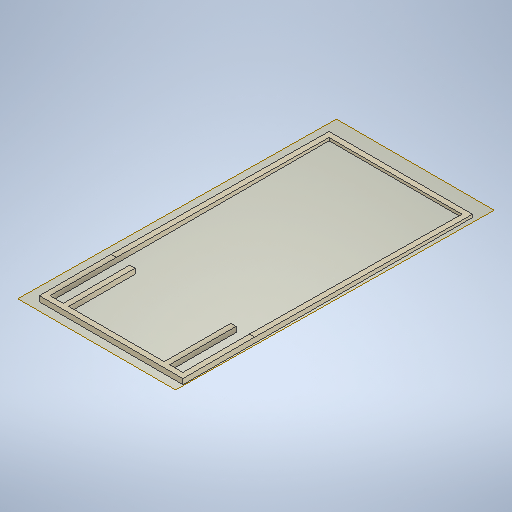
# Autodesk Inventor part: wing1.1
Saved by Autodesk Inventor 2025 (Build 290162000, 162)
## iProperties
Created: 2026-07-27
Part Number: wing1.1
Material: Generic
Document SubType Name: Modeling
Designer: DSTJOHN
Density: 1 g/cm^3
Appearance: Default
Author: DSTJOHN
Autodesk Inventor part; units mm, degrees
ref_plane "YZ Plane" through (0, 0, 0) normal (1, 0, 0) x (0, 1, 0)
ref_plane "XZ Plane" through (0, 0, 0) normal (0, 1, 0) x (-1, 0, 0)
ref_plane "XY Plane" through (0, 0, 0) normal (0, 0, 1) x (1, 0, 0)
sketch "Sketch1" plane through (0, 0, 0) normal (0, 1, 0) x (-1, 0, 0)
  line L0 (0, 0) -> (-50, 0)
  line L1 (-50, 0) -> (-50, -105)
  line L2 (-50, -105) -> (0, -105)
  line L3 (0, -105) -> (0, 0)
  line L4 (2, 2) -> (-52, 2)
  line L5 (-52, 2) -> (-52, -107)
  line L6 (-52, -107) -> (2, -107)
  line L7 (2, -107) -> (2, 2)
  dimension "d0" = 50
  dimension "d1" = 105
  constraints: 16 end point, 4 parallel, 2 horizontal, 2 perpendicular
  measures "d0" distance between parallel lines of L1 L3
  measures "d1" distance between parallel lines of L2 L0
extrude "Extrusion1" add sketch "Sketch1" along normal blind 2
sketch "Sketch2" plane through (0, 2, 0) normal (0, 1, 0) x (1, 0, 0)
  line L0 (0, 0) -> (0, 105) construction
  line L1 (0, 25) -> (50, 25) construction
  line L2 (50, 105) -> (50, 0) construction
  line L3 (0, 105) -> (50, 105) construction
  line L4 (50, 0) -> (0, 0) projected
  line L5 (45, 0) -> (45, 25)
  line L6 (43, 0) -> (43, 25)
  line L7 (5, 0) -> (5, 25)
  line L8 (7, 0) -> (7, 25)
  line L9 (5, 25) -> (7, 25)
  line L10 (5, 0) -> (7, 0)
  line L11 (43, 25) -> (45, 25)
  line L12 (43, 0) -> (45, 0)
  point P0 (25, 105)
  point P1 (5, 12.5)
  dimension "d6" = 80
  dimension "d7" = 5
  dimension "d8" = 2
  dimension "d9" = 5
  dimension "d10" = 2
  constraints: 18 end point, 9 point on line, 4 collinear, 4 perpendicular, 2 midpoint, 1 horizontal
  measures "d6" distance from line of point (25, 105) L1
  measures "d7" distance between parallel lines of L5 L2
  measures "d8" distance between parallel lines of L6 L5
  measures "d9" distance between parallel lines of L7 L0
  measures "d10" distance from line of point (5, 12.5) L8
extrude "Extrusion2" add sketch "Sketch2" against normal blind 2
ref_plane "Work Plane1" through (45, 2, -25) normal (0, 0.9999316, -0.0116934) x (-1, 0, 0)
sketch "Sketch3" plane through (45, 2, -25) normal (0, 0.9999316, -0.0116934) x (-1, 0, 0)
  line L0 (51, 33) -> (-14, 33)
  line L1 (-14, 33) -> (-14, -92)
  line L2 (-14, -92) -> (51, -92)
  line L3 (51, -92) -> (51, 33)
  point P0 (45, 24.9749)
  constraints: 8 end point, 2 parallel, 1 horizontal, 1 perpendicular
extrude "Extrusion3" cut sketch "Sketch3" along normal blind 2
body "Solid1"
